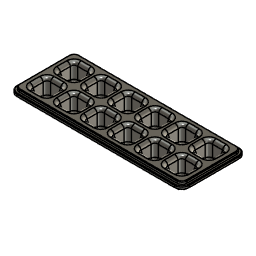
IceCube (Autodesk Fusion 360 design; units mm, degrees)
part number: 2025-04-19-15-41-45-673
part number: 2025-04-19-15-42-12-455
Autodesk Fusion 360 part; units mm, degrees
sketch "Sketch1" plane through (0, 0, 0) normal (0, 0, 1) x (1, 0, 0) in component "cube"
  line L0 (0, 0) -> (13.14, 0)
  line L1 (13.14, 0) -> (13.14, 4.42)
  line L2 (13.14, 4.42) -> (0, 4.42)
  line L3 (0, 4.42) -> (0, 0)
  dimension "d1" = 13.14
  dimension "d2" = 4.42
  constraint horizontal L0
  constraint vertical L1
  constraint horizontal L2
  constraint vertical L3
  constraint coincident L0.start L3.end
  measures "d1" distance of L0.start L0.end
  measures "d2" distance of L0.start L2.end
extrude "Extrude1" add sketch "Sketch1" along normal blind 1.7 in component "cube"
sketch "Sketch2" plane through (0, 0, 1.7) normal (0, 0, 1) x (-1, 0, 0) in component "cube"
  line L0 (0, -4.42) -> (0, 0)
  line L1 (0, 0) -> (-13.14, 0)
  line L2 (-13.14, 0) -> (-13.14, -4.42)
  line L3 (-13.14, -4.42) -> (0, -4.42)
  line L4 (-0.36, -4.06) -> (-1.85, -4.06)
  line L5 (-1.85, -4.06) -> (-1.85, -2.57)
  line L6 (-1.85, -2.57) -> (-0.36, -2.57)
  line L7 (-0.36, -2.57) -> (-0.36, -4.06)
  dimension "d5" = 1.49
  dimension "d6" = 1.49
  dimension "d7" = 0.36
  dimension "d8" = 0.36
  constraint horizontal L4
  constraint vertical L5
  constraint horizontal L6
  constraint vertical L7
  measures "d5" distance of L4.start L4.end
  measures "d6" distance of L4.start L6.end
  measures "d7" distance of L3 L4
  measures "d8" distance of L0 L7
extrude "Extrude2" cut sketch "Sketch2" against normal blind 1.3 draft -10 contours L4 L5 L6 L7 in component "cube"
fillet "Fillet1" radius 0.3 1 edges at (1.105, 2.57, 1.7) 5 faces at (0.9331, 3.4869, 0.4) (1.7736, 3.4869, 1.2667) (0.9331, 3.9836, 1.2667) (0.4364, 3.1431, 1.2667) (1.2769, 2.6464, 1.2667) in component "cube"
pattern_linear "R-Pattern1" count 2 spacing 2.2 along (0, -1, 0) count 6 spacing 2.18 along (1, 0, 0) of "Extrude2", "Fillet1" in component "cube"
shell "Shell1" thickness 0.15 removed faces 5 at (8.76, 4.42, 0.5667) at (13.14, 1.4733, 0.5667) at (4.38, 0, 0.5667) at (0, 2.9467, 0.5667) at (8.76, 1.4733, 0) in component "cube"
fillet "Fillet2" radius 0.2 4 edges at (0, 4.42, 1.625) (0, 0, 1.625) (13.14, 0, 1.625) (13.14, 4.42, 1.625) in component "cube"
ref_plane "WorkPlane1" through (6.57, 2.21, 1.625) normal (0, -1, 0) x (1, 0, 0) in component "cube"
sketch "Sketch3" plane through (0, 2.21, 0) normal (0, -1, 0) x (-1, 0, 0) in component "cube"
  line L0 (0, -1.7) -> (0.2, -1.7)
  line L1 (0.2, -1.7) -> (0.2, -1.5)
  line L2 (0.2, -1.5) -> (0.4, -1.5)
  line L3 (0.4, -1.5) -> (0.4, -1.3)
  line L4 (0.4, -1.3) -> (0, -1.3)
  line L5 (0, -1.3) -> (0, -1.7)
  point P0 (0, -1.7)
  dimension "d20" = 0.2
  dimension "d21" = 0.4
  dimension "d22" = 0.4
  dimension "d23" = 0.2
  constraint horizontal L0
  constraint perpendicular L0 L1
  constraint perpendicular L1 L2
  constraint perpendicular L2 L3
  constraint perpendicular L1 L4
  constraint perpendicular L0 L5
  constraint coincident P0 L0.start
  measures "d20" distance of P0 L0.end
  measures "d21" distance of P0 L4.end
  measures "d22" distance of L3.end L4.end
  measures "d23" distance of L0.end L1.end
sweep "Sweep1" add profiles "Sketch3" along 8 edges at (13.14, 2.21, 1.7) (13.0814, 4.3614, 1.7) (6.57, 4.42, 1.7) (0.0586, 4.3614, 1.7) (0, 2.21, 1.7) (0.0586, 0.0586, 1.7) (6.57, 0, 1.7) (13.0814, 0.0586, 1.7) section 1 in component "cube"
fillet "Fillet3" radius 0.05 16 edges at (6.57, 4.62, 1.7) (-0.0828, 4.5028, 1.7) (-0.2, 2.21, 1.7) (-0.0828, -0.0828, 1.7) (6.57, -0.2, 1.7) (13.2228, -0.0828, 1.7) (13.34, 2.21, 1.7) (13.2228, 4.5028, 1.7) (6.57, 4.82, 1.5) (-0.2243, 4.6443, 1.5) (-0.4, 2.21, 1.5) (-0.2243, -0.2243, 1.5) (6.57, -0.4, 1.5) (13.3643, -0.2243, 1.5) (13.54, 2.21, 1.5) (13.3643, 4.6443, 1.5) in component "cube"
component "cube" placed x (1, 0, 0) y (0, 1, 0) z (0, 0, 1) at (0, 0, 0)
